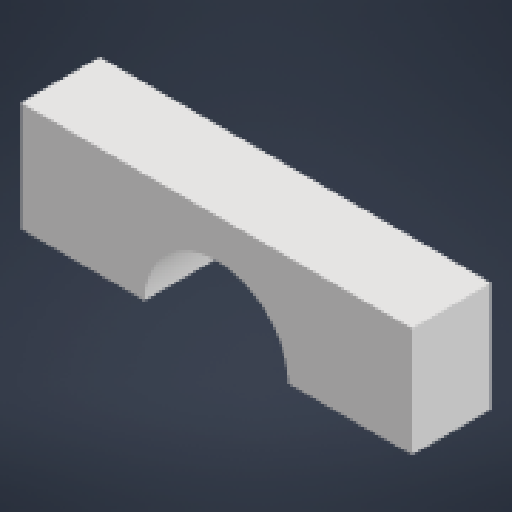
# Autodesk Inventor part: pylon_actuator_holder_jaw
Saved by Autodesk Inventor 2023.2 (Build 272271000, 271)
## iProperties
Created: 2023-07-02
Part Number: pylon_actuator_holder_jaw
Material: Generic
Document SubType Name: Modeling
Designer: Bober
Density: 1 g/cm^3
Appearance: Default
Author: Bober
Autodesk Inventor part; units mm, degrees
ref_plane "YZ Plane" through (0, 0, 0) normal (1, 0, 0) x (0, 1, 0)
ref_plane "XZ Plane" through (0, 0, 0) normal (0, 1, 0) x (-1, 0, 0)
sketch "Sketch1" plane through (0, 0, 0) normal (0, 0, 1) x (1, 0, 0)
  line L0 (-14.8291, -4.1038) -> (-14.8291, 4.1962)
  line L1 (-14.8291, -4.1038) -> (-5.4491, -4.1038)
  arc A0 (5.4491, -4.1038) -> (-5.4491, -4.1038) centre (0, -4.2038) ccw
  line L2 (5.4491, -4.1038) -> (14.8291, -4.1038)
  line L3 (14.8291, -4.1038) -> (14.8291, 4.1962)
  line L4 (-14.8291, 4.1962) -> (14.8291, 4.1962)
  constraints: 10 end point, 2 point on circle, 1 centre point
ref_plane "Work Plane1" through (-18.034, -15.556, -6) normal (0, 0, -1) x (0, 1, 0)
extrude "Extrusion1" add sketch "Sketch1" against normal up to surface (6 mm away)
sketch "Sketch2" plane through (-14.8291, 4.1962, 0) normal (0, 1, 0) x (1, 0, 0)
  circle A0 centre (4, 3) radius 1.5 projected
  circle A1 centre (25.6582, 3) radius 1.5 projected
  point P0 (14.8291, 0)
extrude "Extrusion2" cut sketch "Sketch2" against normal through all
body "Solid1"
